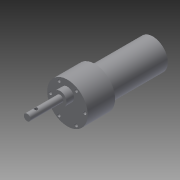
# Autodesk Inventor part: offcentered_shaft_dc_and_encoder
Saved by Autodesk Inventor 2015 (Build 190159000, 159)
## iProperties
Created: 2017-09-26
Part Number: offcentered_shaft_dc_and_encoder
Material: Generic
Document SubType Name: Modeling
Designer: Anshul
Density: 1 g/cm^3
Appearance: Default
Author: Anshul
Autodesk Inventor part; units mm, degrees
ref_plane "YZ Plane" through (0, 0, 0) normal (1, 0, 0) x (0, 1, 0)
ref_plane "XZ Plane" through (0, 0, 0) normal (0, 1, 0) x (-1, 0, 0)
ref_plane "XY Plane" through (0, 0, 0) normal (0, 0, 1) x (1, 0, 0)
sketch "Sketch1" plane through (0, 0, 0) normal (0, 1, 0) x (-1, 0, 0)
  line L0 (0, 0) -> (18.5, 0)
  line L1 (37, 0) -> (37, -25)
  line L2 (0, -25) -> (0, 0)
  line L3 (18.5, -25) -> (18.5, -78)
  line L4 (32.2, -78) -> (32.2, -25)
  line L5 (4.8, -78) -> (4.8, -25)
  line L6 (32.2, -78) -> (4.8, -78)
  line L7 (18.5, -78) -> (18.5, 0)
  line L8 (37, -25) -> (32.2, -25)
  line L9 (18.5, -25) -> (0, -25)
  line L10 (18.5, -25) -> (4.8, -25)
  line L11 (18.5, -78) -> (4.8, -78)
  line L12 (18.5, 0) -> (25.5, 0)
  line L13 (18.5, 0) -> (18.5, 36.8)
  line L14 (18.5, 36.8) -> (18.5, 28.8)
  circle A0 centre (18.5, 28.8) radius 1.5
  dimension "d1" = 25
  dimension "d2" = 53
  dimension "d30" = 36.8
  dimension "d31" = 8
  dimension "d32" = 3
  constraints: 30 end point, 10 perpendicular, 3 horizontal, 3 point on line, 3 vertical, 2 coincident, 1 centre point
  measures "d1" distance of L1.start L1.end
  measures "d2" distance of L3.start L3.end
  measures "d30" distance of L0.end L13.end
  measures "d31" distance of L13.end L14.end
  measures "d32" diameter of A0
revolve "Revolution1" add sketch "Sketch1" angle 360 about axis through (-18.5, 0, -78) along (0, 0, 1) contours L0 L7 L9 L2 | L3 L6 L5 L9
sketch "Sketch2" plane through (-18.5, 0, 0) normal (0, 0, 1) x (1, 0, 0)
  circle A0 centre (0, 0) radius 15.75
  circle A1 centre (-15.75, 0) radius 1.5
  circle A2 centre (15.75, 0) radius 1.5
  line L0 (0, 0) -> (0, 7)
  circle A3 centre (0, 7) radius 6
  circle A4 centre (0, 7) radius 3
  circle A5 centre (-7.875, 13.6399) radius 1.5
  circle A6 centre (7.875, 13.6399) radius 1.5
  circle A7 centre (-7.875, -13.6399) radius 1.5
  circle A8 centre (7.875, -13.6399) radius 1.5
  point P0 (18.5, 0)
  dimension "d12" = 3
  dimension "d13" = 3
  dimension "d14" = 7
  dimension "d15" = 12
  dimension "d16" = 6
  dimension "d17" = 3
  dimension "d18" = 3
  dimension "d19" = 3
  dimension "d20" = 3
  constraints: 9 centre point, 6 point on circle, 2 coincident, 2 end point, 1 vertical
  measures "d12" diameter of A1
  measures "d13" diameter of A2
  measures "d14" distance of L0.start L0.end
  measures "d15" diameter of A3
  measures "d16" diameter of A4
  measures "d17" diameter of A5
  measures "d18" diameter of A6
  measures "d19" diameter of A7
  measures "d20" diameter of A8
extrude "Extrusion3" add sketch "Sketch2" along normal blind 6.8 contours A3
extrude "Extrusion4" add sketch "Sketch2" along normal blind 36.8 contours A4
extrude "Extrusion5" cut sketch "Sketch2" against normal blind 5 contours A0 A2 | A0 A2 | A6 A0 | A0 A6 | A8 A0 | A0 A8 | A5 A0 | A0 A5 | A7 A0 | A0 A7 | A1 A0 | A0 A1
extrude "Extrusion6" cut sketch "Sketch1" along normal blind 20 contours A0 L13 | L13 A0
body "Solid1"
